Autodesk Inventor part; units mm, degrees
note: some values were not read from the file. Chosen so that the rebuilt part matches the saved one: direction of "Emboss1".
(part 2 of 2)
sketch "Sketch6" plane through (0, 0, 0) normal (0, 0, -1) x (-1, 0, 0)
  line L0 (6.1173, 8.8105) -> (-5.4561, 8.8105) construction
  line L1 (-5.4561, 8.8105) -> (-5.4561, 10.3737) construction
  line L2 (-5.4561, 10.3737) -> (6.1173, 10.3737) construction
  line L3 (6.1173, 10.3737) -> (6.1173, 8.8105) construction
  line L4 (-8.9202, 5.2044) -> (-8.9202, -5.2664) construction
  line L5 (-8.9202, -5.2664) -> (-10.8128, -5.2664) construction
  line L6 (-10.8128, -5.2664) -> (-10.8128, 5.2044) construction
  line L7 (-10.8128, 5.2044) -> (-8.9202, 5.2044) construction
  line L8 (5.1582, 10.3421) -> (5.89, 10.3421)
  line L9 (5.89, 10.3421) -> (5.89, 10.1889)
  line L10 (5.89, 10.1889) -> (5.6177, 10.1889)
  line L11 (5.6177, 10.1889) -> (5.6177, 9.1837)
  line L12 (5.6177, 9.1837) -> (5.89, 9.1837)
  line L13 (5.89, 9.1837) -> (5.89, 9.0463)
  spline S0 degree 2 poles (5.89, 9.0463) (5.7356, 9.0463) (5.5897, 8.9588) (5.58, 8.8372) knots 0 0 0 1 2 2 2
  line L14 (5.58, 8.8372) -> (5.4244, 8.8372)
  line L15 (5.4244, 8.8372) -> (5.4244, 10.1889)
  line L16 (5.4244, 10.1889) -> (5.1582, 10.1889)
  line L17 (5.1582, 10.1889) -> (5.1582, 10.3421)
  spline S1 degree 2 poles (3.9487, 9.5921) (3.9487, 9.9957) (4.1833, 10.3737) (4.4277, 10.3737) knots 0 0 0 1 2 2 2
  spline S2 degree 2 poles (4.4277, 10.3737) (4.6756, 10.3737) (4.9078, 9.9884) (4.9078, 9.5933) knots 0 0 0 1 2 2 2
  spline S3 degree 2 poles (4.9078, 9.5933) (4.9078, 9.1873) (4.6732, 8.8117) (4.4277, 8.8117) knots 0 0 0 1 2 2 2
  spline S4 degree 2 poles (4.4277, 8.8117) (4.1809, 8.8117) (3.9487, 9.2007) (3.9487, 9.5921) knots 0 0 0 1 2 2 2
  spline S5 degree 2 poles (4.2064, 10.0491) (4.1773, 9.975) (4.1529, 9.7465) (4.1529, 9.5921) knots 0 0 0 1 2 2 2
  spline S6 degree 2 poles (4.1529, 9.5921) (4.1529, 9.4377) (4.1773, 9.2104) (4.2076, 9.1338) knots 0 0 0 1 2 2 2
  spline S7 degree 2 poles (4.2076, 9.1338) (4.238, 9.0572) (4.3438, 8.9782) (4.4277, 8.9782) knots 0 0 0 1 2 2 2
  spline S8 degree 2 poles (4.4277, 8.9782) (4.5115, 8.9782) (4.6197, 9.0572) (4.6513, 9.1362) knots 0 0 0 1 2 2 2
  spline S9 degree 2 poles (4.6513, 9.1362) (4.6817, 9.2128) (4.7036, 9.4462) (4.7036, 9.5933) knots 0 0 0 1 2 2 2
  spline S10 degree 2 poles (4.7036, 9.5933) (4.7036, 9.7513) (4.6841, 9.9628) (4.6525, 10.0455) knots 0 0 0 1 2 2 2
  spline S11 degree 2 poles (4.6525, 10.0455) (4.6234, 10.1233) (4.5152, 10.2072) (4.4277, 10.2072) knots 0 0 0 1 2 2 2
  spline S12 degree 2 poles (4.4277, 10.2072) (4.345, 10.2072) (4.2368, 10.1281) (4.2064, 10.0491) knots 0 0 0 1 2 2 2
  line L18 (2.5533, 10.3421) -> (2.8122, 10.3421)
  line L19 (2.8122, 10.3421) -> (3.2862, 9.7452)
  line L20 (3.2862, 9.7452) -> (3.5148, 9.7452)
  line L21 (3.5148, 9.7452) -> (3.5148, 10.3421)
  line L22 (3.5148, 10.3421) -> (3.7141, 10.3421)
  line L23 (3.7141, 10.3421) -> (3.7141, 8.8421)
  line L24 (3.7141, 8.8421) -> (3.3276, 8.8421)
  spline S13 degree 2 poles (3.3276, 8.8421) (3.1987, 8.8421) (3.0249, 8.87) (2.9459, 8.9211) knots 0 0 0 1 2 2 2
  spline S14 degree 2 poles (2.9459, 8.9211) (2.8669, 8.9721) (2.7757, 9.1314) (2.7757, 9.2493) knots 0 0 0 1 2 2 2
  spline S15 degree 2 poles (2.7757, 9.2493) (2.7757, 9.4134) (2.9435, 9.6358) (3.0869, 9.6893) knots 0 0 0 1 2 2 2
  line L25 (3.0869, 9.6893) -> (2.5533, 10.3421)
  spline S16 degree 2 poles (2.9836, 9.2651) (2.9836, 9.1995) (3.0298, 9.0986) (3.0784, 9.0657) knots 0 0 0 1 2 2 2
  spline S17 degree 2 poles (3.0784, 9.0657) (3.1209, 9.0378) (3.234, 9.0147) (3.3166, 9.0147) knots 0 0 0 1 2 2 2
  line L26 (3.3166, 9.0147) -> (3.5148, 9.0147)
  line L27 (3.5148, 9.0147) -> (3.5148, 9.5787)
  line L28 (3.5148, 9.5787) -> (3.3397, 9.5787)
  spline S18 degree 2 poles (3.3397, 9.5787) (3.2534, 9.5787) (3.1161, 9.5483) (3.0687, 9.5009) knots 0 0 0 1 2 2 2
  spline S19 degree 2 poles (3.0687, 9.5009) (3.0249, 9.4596) (2.9836, 9.3429) (2.9836, 9.2651) knots 0 0 0 1 2 2 2
  spline S20 degree 2 poles (0.8989, 9.5921) (0.8989, 9.9957) (1.1335, 10.3737) (1.3778, 10.3737) knots 0 0 0 1 2 2 2
  spline S21 degree 2 poles (1.3778, 10.3737) (1.6258, 10.3737) (1.858, 9.9884) (1.858, 9.5933) knots 0 0 0 1 2 2 2
  spline S22 degree 2 poles (1.858, 9.5933) (1.858, 9.1873) (1.6234, 8.8117) (1.3778, 8.8117) knots 0 0 0 1 2 2 2
  spline S23 degree 2 poles (1.3778, 8.8117) (1.1311, 8.8117) (0.8989, 9.2007) (0.8989, 9.5921) knots 0 0 0 1 2 2 2
  spline S24 degree 2 poles (1.1566, 10.0491) (1.1274, 9.975) (1.1031, 9.7465) (1.1031, 9.5921) knots 0 0 0 1 2 2 2
  spline S25 degree 2 poles (1.1031, 9.5921) (1.1031, 9.4377) (1.1274, 9.2104) (1.1578, 9.1338) knots 0 0 0 1 2 2 2
  spline S26 degree 2 poles (1.1578, 9.1338) (1.1882, 9.0572) (1.2939, 8.9782) (1.3778, 8.9782) knots 0 0 0 1 2 2 2
  spline S27 degree 2 poles (1.3778, 8.9782) (1.4617, 8.9782) (1.5699, 9.0572) (1.6015, 9.1362) knots 0 0 0 1 2 2 2
  spline S28 degree 2 poles (1.6015, 9.1362) (1.6319, 9.2128) (1.6537, 9.4462) (1.6537, 9.5933) knots 0 0 0 1 2 2 2
  spline S29 degree 2 poles (1.6537, 9.5933) (1.6537, 9.7513) (1.6343, 9.9628) (1.6027, 10.0455) knots 0 0 0 1 2 2 2
  spline S30 degree 2 poles (1.6027, 10.0455) (1.5735, 10.1233) (1.4653, 10.2072) (1.3778, 10.2072) knots 0 0 0 1 2 2 2
  spline S31 degree 2 poles (1.3778, 10.2072) (1.2952, 10.2072) (1.187, 10.1281) (1.1566, 10.0491) knots 0 0 0 1 2 2 2
  line L29 (-0.2182, 10.3421) -> (0.7068, 10.3421)
  line L30 (0.7068, 10.3421) -> (0.7068, 10.1294)
  spline S32 degree 2 poles (0.7068, 10.1294) (0.6072, 10.0358) (0.4297, 9.8619) (0.3446, 9.7683) knots 0 0 0 1 2 2 2
  spline S33 degree 2 poles (0.3446, 9.7683) (0.1732, 9.5799) (0.048, 9.3538) (0.048, 9.2335) knots 0 0 0 1 2 2 2
  spline S34 degree 2 poles (0.048, 9.2335) (0.048, 9.1703) (0.0869, 9.0755) (0.1221, 9.0451) knots 0 0 0 1 2 2 2
  spline S35 degree 2 poles (0.1221, 9.0451) (0.1574, 9.0147) (0.2498, 8.9843) (0.3057, 8.9843) knots 0 0 0 1 2 2 2
  spline S36 degree 2 poles (0.3057, 8.9843) (0.3592, 8.9843) (0.4686, 9.011) (0.5184, 9.0317) knots 0 0 0 1 2 2 2
  spline S37 degree 2 poles (0.5184, 9.0317) (0.561, 9.0487) (0.64, 9.0974) (0.6643, 9.1144) knots 0 0 0 1 2 2 2
  line L31 (0.6643, 9.1144) -> (0.6752, 9.1144)
  line L32 (0.6752, 9.1144) -> (0.6752, 8.9004)
  spline S38 degree 2 poles (0.6752, 8.9004) (0.6132, 8.87) (0.3908, 8.8105) (0.2911, 8.8105) knots 0 0 0 1 2 2 2
  spline S39 degree 2 poles (0.2911, 8.8105) (0.0808, 8.8105) (-0.1562, 9.0329) (-0.1562, 9.2226) knots 0 0 0 1 2 2 2
  spline S40 degree 2 poles (-0.1562, 9.2226) (-0.1562, 9.3113) (-0.1149, 9.4596) (-0.0784, 9.5228) knots 0 0 0 1 2 2 2
  spline S41 degree 2 poles (-0.0784, 9.5228) (-0.042, 9.5884) (0.0638, 9.7173) (0.1221, 9.7793) knots 0 0 0 1 2 2 2
  spline S42 degree 2 poles (0.1221, 9.7793) (0.217, 9.8826) (0.4491, 10.1038) (0.5184, 10.1683) knots 0 0 0 1 2 2 2
  line L33 (0.5184, 10.1683) -> (-0.2182, 10.1683)
  line L34 (-0.2182, 10.1683) -> (-0.2182, 10.3421)
  line L35 (-2.0051, 9.067) -> (-1.356, 10.3421)
  line L36 (-1.356, 10.3421) -> (-1.142, 10.3421)
  line L37 (-1.142, 10.3421) -> (-1.8276, 9.0183)
  line L38 (-1.8276, 9.0183) -> (-1.0533, 9.0183)
  line L39 (-1.0533, 9.0183) -> (-1.0533, 8.8421)
  line L40 (-1.0533, 8.8421) -> (-2.0051, 8.8421)
  line L41 (-2.0051, 8.8421) -> (-2.0051, 9.067)
  spline S43 degree 2 poles (-3.1222, 9.5921) (-3.1222, 9.9957) (-2.8876, 10.3737) (-2.6433, 10.3737) knots 0 0 0 1 2 2 2
  spline S44 degree 2 poles (-2.6433, 10.3737) (-2.3953, 10.3737) (-2.1631, 9.9884) (-2.1631, 9.5933) knots 0 0 0 1 2 2 2
  spline S45 degree 2 poles (-2.1631, 9.5933) (-2.1631, 9.1873) (-2.3977, 8.8117) (-2.6433, 8.8117) knots 0 0 0 1 2 2 2
  spline S46 degree 2 poles (-2.6433, 8.8117) (-2.89, 8.8117) (-3.1222, 9.2007) (-3.1222, 9.5921) knots 0 0 0 1 2 2 2
  spline S47 degree 2 poles (-2.8645, 10.0491) (-2.8937, 9.975) (-2.918, 9.7465) (-2.918, 9.5921) knots 0 0 0 1 2 2 2
  spline S48 degree 2 poles (-2.918, 9.5921) (-2.918, 9.4377) (-2.8937, 9.2104) (-2.8633, 9.1338) knots 0 0 0 1 2 2 2
  spline S49 degree 2 poles (-2.8633, 9.1338) (-2.8329, 9.0572) (-2.7271, 8.9782) (-2.6433, 8.9782) knots 0 0 0 1 2 2 2
  spline S50 degree 2 poles (-2.6433, 8.9782) (-2.5594, 8.9782) (-2.4512, 9.0572) (-2.4196, 9.1362) knots 0 0 0 1 2 2 2
  spline S51 degree 2 poles (-2.4196, 9.1362) (-2.3892, 9.2128) (-2.3673, 9.4462) (-2.3673, 9.5933) knots 0 0 0 1 2 2 2
  spline S52 degree 2 poles (-2.3673, 9.5933) (-2.3673, 9.7513) (-2.3868, 9.9628) (-2.4184, 10.0455) knots 0 0 0 1 2 2 2
  spline S53 degree 2 poles (-2.4184, 10.0455) (-2.4475, 10.1233) (-2.5557, 10.2072) (-2.6433, 10.2072) knots 0 0 0 1 2 2 2
  spline S54 degree 2 poles (-2.6433, 10.2072) (-2.7259, 10.2072) (-2.8341, 10.1281) (-2.8645, 10.0491) knots 0 0 0 1 2 2 2
  line L42 (-4.2393, 10.3421) -> (-3.3142, 10.3421)
  line L43 (-3.3142, 10.3421) -> (-3.3142, 10.1294)
  spline S55 degree 2 poles (-3.3142, 10.1294) (-3.4139, 10.0358) (-3.5914, 9.8619) (-3.6765, 9.7683) knots 0 0 0 1 2 2 2
  spline S56 degree 2 poles (-3.6765, 9.7683) (-3.8479, 9.5799) (-3.9731, 9.3538) (-3.9731, 9.2335) knots 0 0 0 1 2 2 2
  spline S57 degree 2 poles (-3.9731, 9.2335) (-3.9731, 9.1703) (-3.9342, 9.0755) (-3.8989, 9.0451) knots 0 0 0 1 2 2 2
  spline S58 degree 2 poles (-3.8989, 9.0451) (-3.8637, 9.0147) (-3.7713, 8.9843) (-3.7154, 8.9843) knots 0 0 0 1 2 2 2
  spline S59 degree 2 poles (-3.7154, 8.9843) (-3.6619, 8.9843) (-3.5525, 9.011) (-3.5027, 9.0317) knots 0 0 0 1 2 2 2
  spline S60 degree 2 poles (-3.5027, 9.0317) (-3.4601, 9.0487) (-3.3811, 9.0974) (-3.3568, 9.1144) knots 0 0 0 1 2 2 2
  line L44 (-3.3568, 9.1144) -> (-3.3458, 9.1144)
  line L45 (-3.3458, 9.1144) -> (-3.3458, 8.9004)
  spline S61 degree 2 poles (-3.3458, 8.9004) (-3.4078, 8.87) (-3.6303, 8.8105) (-3.73, 8.8105) knots 0 0 0 1 2 2 2
  spline S62 degree 2 poles (-3.73, 8.8105) (-3.9403, 8.8105) (-4.1773, 9.0329) (-4.1773, 9.2226) knots 0 0 0 1 2 2 2
  spline S63 degree 2 poles (-4.1773, 9.2226) (-4.1773, 9.3113) (-4.136, 9.4596) (-4.0995, 9.5228) knots 0 0 0 1 2 2 2
  spline S64 degree 2 poles (-4.0995, 9.5228) (-4.063, 9.5884) (-3.9573, 9.7173) (-3.8989, 9.7793) knots 0 0 0 1 2 2 2
  spline S65 degree 2 poles (-3.8989, 9.7793) (-3.8041, 9.8826) (-3.5719, 10.1038) (-3.5027, 10.1683) knots 0 0 0 1 2 2 2
  line L46 (-3.5027, 10.1683) -> (-4.2393, 10.1683)
  line L47 (-4.2393, 10.1683) -> (-4.2393, 10.3421)
  spline S66 degree 2 poles (-5.3491, 9.8656) (-5.3491, 9.9738) (-5.2798, 10.1585) (-5.2166, 10.2266) knots 0 0 0 1 2 2 2
  spline S67 degree 2 poles (-5.2166, 10.2266) (-5.1534, 10.2947) (-4.965, 10.3737) (-4.8483, 10.3737) knots 0 0 0 1 2 2 2
  spline S68 degree 2 poles (-4.8483, 10.3737) (-4.7413, 10.3737) (-4.5322, 10.3263) (-4.4557, 10.2886) knots 0 0 0 1 2 2 2
  line L48 (-4.4557, 10.2886) -> (-4.4557, 10.0759)
  line L49 (-4.4557, 10.0759) -> (-4.4702, 10.0759)
  spline S69 degree 2 poles (-4.4702, 10.0759) (-4.4933, 10.0929) (-4.5796, 10.1367) (-4.6319, 10.1561) knots 0 0 0 1 2 2 2
  spline S70 degree 2 poles (-4.6319, 10.1561) (-4.6915, 10.1768) (-4.7899, 10.1999) (-4.8519, 10.1999) knots 0 0 0 1 2 2 2
  spline S71 degree 2 poles (-4.8519, 10.1999) (-4.9127, 10.1999) (-5.027, 10.1561) (-5.0683, 10.1087) knots 0 0 0 1 2 2 2
  spline S72 degree 2 poles (-5.0683, 10.1087) (-5.106, 10.0637) (-5.1449, 9.9446) (-5.1449, 9.8644) knots 0 0 0 1 2 2 2
  spline S73 degree 2 poles (-5.1449, 9.8644) (-5.1449, 9.7841) (-5.1011, 9.682) (-5.0598, 9.648) knots 0 0 0 1 2 2 2
  spline S74 degree 2 poles (-5.0598, 9.648) (-5.0172, 9.6103) (-4.8908, 9.5787) (-4.8142, 9.5787) knots 0 0 0 1 2 2 2
  spline S75 degree 2 poles (-4.8142, 9.5787) (-4.7316, 9.5787) (-4.5675, 9.6042) (-4.5176, 9.6152) knots 0 0 0 1 2 2 2
  line L50 (-4.5176, 9.6152) -> (-4.5176, 8.8421)
  line L51 (-4.5176, 8.8421) -> (-5.3406, 8.8421)
  line L52 (-5.3406, 8.8421) -> (-5.3406, 9.0183)
  line L53 (-5.3406, 9.0183) -> (-4.7109, 9.0183)
  line L54 (-4.7109, 9.0183) -> (-4.7109, 9.4183)
  spline S76 degree 2 poles (-4.7109, 9.4183) (-4.7474, 9.4134) (-4.8179, 9.4098) (-4.8471, 9.4098) knots 0 0 0 1 2 2 2
  spline S77 degree 2 poles (-4.8471, 9.4098) (-4.9625, 9.4098) (-5.1218, 9.4474) (-5.1947, 9.5033) knots 0 0 0 1 2 2 2
  spline S78 degree 2 poles (-5.1947, 9.5033) (-5.2689, 9.5593) (-5.3491, 9.7294) (-5.3491, 9.8656) knots 0 0 0 1 2 2 2
  line L55 (-10.4871, 4.17) -> (-10.4871, 5.095)
  line L56 (-10.4871, 5.095) -> (-10.2743, 5.095)
  spline S79 degree 2 poles (-10.2743, 5.095) (-10.1807, 4.9954) (-10.0069, 4.8179) (-9.9133, 4.7328) knots 0 0 0 1 2 2 2
  spline S80 degree 2 poles (-9.9133, 4.7328) (-9.7249, 4.5614) (-9.4988, 4.4362) (-9.3785, 4.4362) knots 0 0 0 1 2 2 2
  spline S81 degree 2 poles (-9.3785, 4.4362) (-9.3153, 4.4362) (-9.2205, 4.4751) (-9.1901, 4.5104) knots 0 0 0 1 2 2 2
  spline S82 degree 2 poles (-9.1901, 4.5104) (-9.1597, 4.5456) (-9.1293, 4.638) (-9.1293, 4.6939) knots 0 0 0 1 2 2 2
  spline S83 degree 2 poles (-9.1293, 4.6939) (-9.1293, 4.7474) (-9.156, 4.8568) (-9.1767, 4.9066) knots 0 0 0 1 2 2 2
  spline S84 degree 2 poles (-9.1767, 4.9066) (-9.1937, 4.9492) (-9.2423, 5.0282) (-9.2594, 5.0525) knots 0 0 0 1 2 2 2
  line L57 (-9.2594, 5.0525) -> (-9.2594, 5.0634)
  line L58 (-9.2594, 5.0634) -> (-9.0454, 5.0634)
  spline S85 degree 2 poles (-9.0454, 5.0634) (-9.015, 5.0014) (-8.9555, 4.779) (-8.9555, 4.6793) knots 0 0 0 1 2 2 2
  spline S86 degree 2 poles (-8.9555, 4.6793) (-8.9555, 4.469) (-9.1779, 4.232) (-9.3675, 4.232) knots 0 0 0 1 2 2 2
  spline S87 degree 2 poles (-9.3675, 4.232) (-9.4563, 4.232) (-9.6046, 4.2733) (-9.6678, 4.3098) knots 0 0 0 1 2 2 2
  spline S88 degree 2 poles (-9.6678, 4.3098) (-9.7334, 4.3463) (-9.8623, 4.452) (-9.9243, 4.5104) knots 0 0 0 1 2 2 2
  spline S89 degree 2 poles (-9.9243, 4.5104) (-10.0276, 4.6052) (-10.2488, 4.8373) (-10.3132, 4.9066) knots 0 0 0 1 2 2 2
  line L59 (-10.3132, 4.9066) -> (-10.3132, 4.17)
  line L60 (-10.3132, 4.17) -> (-10.4871, 4.17)
  line L61 (-9.9717, 3.0043) -> (-9.9717, 3.183)
  line L62 (-9.9717, 3.183) -> (-10.4871, 3.183)
  line L63 (-10.4871, 3.183) -> (-10.4871, 3.3762)
  line L64 (-10.4871, 3.3762) -> (-9.9717, 3.3762)
  line L65 (-9.9717, 3.3762) -> (-9.9717, 4.0387)
  line L66 (-9.9717, 4.0387) -> (-9.7602, 4.0387)
  line L67 (-9.7602, 4.0387) -> (-8.9871, 3.3677)
  line L68 (-8.9871, 3.3677) -> (-8.9871, 3.183)
  line L69 (-8.9871, 3.183) -> (-9.81, 3.183)
  line L70 (-9.81, 3.183) -> (-9.81, 3.0043)
  line L71 (-9.81, 3.0043) -> (-9.9717, 3.0043)
  line L72 (-9.81, 3.3762) -> (-9.2241, 3.3762)
  line L73 (-9.2241, 3.3762) -> (-9.81, 3.8807)
  line L74 (-9.81, 3.8807) -> (-9.81, 3.3762)
  line L75 (-9.3615, 1.9322) -> (-10.4871, 2.3564)
  line L76 (-10.4871, 2.3564) -> (-10.4871, 2.5266)
  line L77 (-10.4871, 2.5266) -> (-9.3615, 2.9471)
  line L78 (-9.3615, 2.9471) -> (-9.3615, 2.7417)
  line L79 (-9.3615, 2.7417) -> (-10.2282, 2.4342)
  line L80 (-10.2282, 2.4342) -> (-9.3615, 2.1291)
  line L81 (-9.3615, 2.1291) -> (-9.3615, 1.9322)
  line L82 (-10.4871, 0.3228) -> (-10.4871, 1.0545)
  line L83 (-10.4871, 1.0545) -> (-10.3339, 1.0545)
  line L84 (-10.3339, 1.0545) -> (-10.3339, 0.7822)
  line L85 (-10.3339, 0.7822) -> (-9.3286, 0.7822)
  line L86 (-9.3286, 0.7822) -> (-9.3286, 1.0545)
  line L87 (-9.3286, 1.0545) -> (-9.1913, 1.0545)
  spline S90 degree 2 poles (-9.1913, 1.0545) (-9.1913, 0.9001) (-9.1038, 0.7543) (-8.9822, 0.7445) knots 0 0 0 1 2 2 2
  line L88 (-8.9822, 0.7445) -> (-8.9822, 0.589)
  line L89 (-8.9822, 0.589) -> (-10.3339, 0.589)
  line L90 (-10.3339, 0.589) -> (-10.3339, 0.3228)
  line L91 (-10.3339, 0.3228) -> (-10.4871, 0.3228)
  spline S91 degree 2 poles (-9.7371, -0.8867) (-10.1406, -0.8867) (-10.5187, -0.6521) (-10.5187, -0.4078) knots 0 0 0 1 2 2 2
  spline S92 degree 2 poles (-10.5187, -0.4078) (-10.5187, -0.1598) (-10.1333, 0.0723) (-9.7383, 0.0723) knots 0 0 0 1 2 2 2
  spline S93 degree 2 poles (-9.7383, 0.0723) (-9.3323, 0.0723) (-8.9567, -0.1623) (-8.9567, -0.4078) knots 0 0 0 1 2 2 2
  spline S94 degree 2 poles (-8.9567, -0.4078) (-8.9567, -0.6546) (-9.3457, -0.8867) (-9.7371, -0.8867) knots 0 0 0 1 2 2 2
  spline S95 degree 2 poles (-10.1941, -0.629) (-10.12, -0.6582) (-9.8914, -0.6825) (-9.7371, -0.6825) knots 0 0 0 1 2 2 2
  spline S96 degree 2 poles (-9.7371, -0.6825) (-9.5827, -0.6825) (-9.3554, -0.6582) (-9.2788, -0.6278) knots 0 0 0 1 2 2 2
  spline S97 degree 2 poles (-9.2788, -0.6278) (-9.2022, -0.5974) (-9.1232, -0.4917) (-9.1232, -0.4078) knots 0 0 0 1 2 2 2
  spline S98 degree 2 poles (-9.1232, -0.4078) (-9.1232, -0.3239) (-9.2022, -0.2157) (-9.2812, -0.1841) knots 0 0 0 1 2 2 2
  spline S99 degree 2 poles (-9.2812, -0.1841) (-9.3578, -0.1537) (-9.5912, -0.1319) (-9.7383, -0.1319) knots 0 0 0 1 2 2 2
  spline S100 degree 2 poles (-9.7383, -0.1319) (-9.8963, -0.1319) (-10.1078, -0.1513) (-10.1905, -0.1829) knots 0 0 0 1 2 2 2
  spline S101 degree 2 poles (-10.1905, -0.1829) (-10.2683, -0.2121) (-10.3521, -0.3203) (-10.3521, -0.4078) knots 0 0 0 1 2 2 2
  spline S102 degree 2 poles (-10.3521, -0.4078) (-10.3521, -0.4905) (-10.2731, -0.5986) (-10.1941, -0.629) knots 0 0 0 1 2 2 2
  line L92 (-8.9202, -1.7024) -> (-10.8128, -1.1153)
  line L93 (-10.8128, -1.1153) -> (-10.8128, -0.9451)
  line L94 (-10.8128, -0.9451) -> (-8.9202, -1.5298)
  line L95 (-8.9202, -1.5298) -> (-8.9202, -1.7024)
  line L96 (-10.4871, -2.7927) -> (-10.4871, -1.8677)
  line L97 (-10.4871, -1.8677) -> (-10.2743, -1.8677)
  spline S103 degree 2 poles (-10.2743, -1.8677) (-10.1807, -1.9674) (-10.0069, -2.1448) (-9.9133, -2.2299) knots 0 0 0 1 2 2 2
  spline S104 degree 2 poles (-9.9133, -2.2299) (-9.7249, -2.4013) (-9.4988, -2.5265) (-9.3785, -2.5265) knots 0 0 0 1 2 2 2
  spline S105 degree 2 poles (-9.3785, -2.5265) (-9.3153, -2.5265) (-9.2205, -2.4876) (-9.1901, -2.4524) knots 0 0 0 1 2 2 2
  spline S106 degree 2 poles (-9.1901, -2.4524) (-9.1597, -2.4171) (-9.1293, -2.3247) (-9.1293, -2.2688) knots 0 0 0 1 2 2 2
  spline S107 degree 2 poles (-9.1293, -2.2688) (-9.1293, -2.2153) (-9.156, -2.1059) (-9.1767, -2.0561) knots 0 0 0 1 2 2 2
  spline S108 degree 2 poles (-9.1767, -2.0561) (-9.1937, -2.0136) (-9.2423, -1.9345) (-9.2594, -1.9102) knots 0 0 0 1 2 2 2
  line L98 (-9.2594, -1.9102) -> (-9.2594, -1.8993)
  line L99 (-9.2594, -1.8993) -> (-9.0454, -1.8993)
  spline S109 degree 2 poles (-9.0454, -1.8993) (-9.015, -1.9613) (-8.9555, -2.1837) (-8.9555, -2.2834) knots 0 0 0 1 2 2 2
  spline S110 degree 2 poles (-8.9555, -2.2834) (-8.9555, -2.4937) (-9.1779, -2.7307) (-9.3675, -2.7307) knots 0 0 0 1 2 2 2
  spline S111 degree 2 poles (-9.3675, -2.7307) (-9.4563, -2.7307) (-9.6046, -2.6894) (-9.6678, -2.6529) knots 0 0 0 1 2 2 2
  spline S112 degree 2 poles (-9.6678, -2.6529) (-9.7334, -2.6165) (-9.8623, -2.5107) (-9.9243, -2.4524) knots 0 0 0 1 2 2 2
  spline S113 degree 2 poles (-9.9243, -2.4524) (-10.0276, -2.3576) (-10.2488, -2.1254) (-10.3132, -2.0561) knots 0 0 0 1 2 2 2
  line L100 (-10.3132, -2.0561) -> (-10.3132, -2.7927)
  line L101 (-10.3132, -2.7927) -> (-10.4871, -2.7927)
  spline S114 degree 2 poles (-9.7371, -3.9268) (-10.1406, -3.9268) (-10.5187, -3.6922) (-10.5187, -3.4479) knots 0 0 0 1 2 2 2
  spline S115 degree 2 poles (-10.5187, -3.4479) (-10.5187, -3.1999) (-10.1333, -2.9678) (-9.7383, -2.9678) knots 0 0 0 1 2 2 2
  spline S116 degree 2 poles (-9.7383, -2.9678) (-9.3323, -2.9678) (-8.9567, -3.2024) (-8.9567, -3.4479) knots 0 0 0 1 2 2 2
  spline S117 degree 2 poles (-8.9567, -3.4479) (-8.9567, -3.6947) (-9.3457, -3.9268) (-9.7371, -3.9268) knots 0 0 0 1 2 2 2
  spline S118 degree 2 poles (-10.1941, -3.6691) (-10.12, -3.6983) (-9.8914, -3.7226) (-9.7371, -3.7226) knots 0 0 0 1 2 2 2
  spline S119 degree 2 poles (-9.7371, -3.7226) (-9.5827, -3.7226) (-9.3554, -3.6983) (-9.2788, -3.6679) knots 0 0 0 1 2 2 2
  spline S120 degree 2 poles (-9.2788, -3.6679) (-9.2022, -3.6375) (-9.1232, -3.5318) (-9.1232, -3.4479) knots 0 0 0 1 2 2 2
  spline S121 degree 2 poles (-9.1232, -3.4479) (-9.1232, -3.364) (-9.2022, -3.2559) (-9.2812, -3.2243) knots 0 0 0 1 2 2 2
  spline S122 degree 2 poles (-9.2812, -3.2243) (-9.3578, -3.1939) (-9.5912, -3.172) (-9.7383, -3.172) knots 0 0 0 1 2 2 2
  spline S123 degree 2 poles (-9.7383, -3.172) (-9.8963, -3.172) (-10.1078, -3.1914) (-10.1905, -3.223) knots 0 0 0 1 2 2 2
  spline S124 degree 2 poles (-10.1905, -3.223) (-10.2683, -3.2522) (-10.3521, -3.3604) (-10.3521, -3.4479) knots 0 0 0 1 2 2 2
  spline S125 degree 2 poles (-10.3521, -3.4479) (-10.3521, -3.5306) (-10.2731, -3.6388) (-10.1941, -3.6691) knots 0 0 0 1 2 2 2
  line L102 (-10.4871, -3.9998) -> (-8.9871, -4.5055)
  line L103 (-8.9871, -4.5055) -> (-8.9871, -4.751)
  line L104 (-8.9871, -4.751) -> (-10.4871, -5.2567)
  line L105 (-10.4871, -5.2567) -> (-10.4871, -5.0464)
  line L106 (-10.4871, -5.0464) -> (-10.0677, -4.9102)
  line L107 (-10.0677, -4.9102) -> (-10.0677, -4.3377)
  line L108 (-10.0677, -4.3377) -> (-10.4871, -4.2016)
  line L109 (-10.4871, -4.2016) -> (-10.4871, -3.9998)
  line L110 (-9.8975, -4.8555) -> (-9.1913, -4.6234)
  line L111 (-9.1913, -4.6234) -> (-9.8975, -4.3924)
  line L112 (-9.8975, -4.3924) -> (-9.8975, -4.8555)
  point P0 (0, 0)
  constraints: 4 other
extrude "Extrusion4" add sketch "Sketch6" along normal blind 0.1
body "Solid1"
